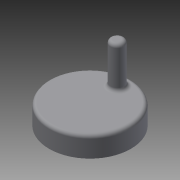
# Autodesk Inventor part: Handle
Saved by Autodesk Inventor 2014 (Build 180170000, 170)
## iProperties
Created: 2014-05-06
Part Number: Handle
Material: Generic
Document SubType Name: Modeling
Designer: Tristan Debrunner
Density: 1 g/cm^3
Appearance: Default
Author: Tristan Debrunner
Autodesk Inventor part; units mm, degrees
ref_plane "YZ Plane" through (0, 0, 0) normal (1, 0, 0) x (0, 1, 0)
ref_plane "XZ Plane" through (0, 0, 0) normal (0, 1, 0) x (-1, 0, 0)
ref_plane "XY Plane" through (0, 0, 0) normal (0, 0, 1) x (1, 0, 0)
sketch "Sketch1" plane through (0, 0, 0) normal (0, 1, 0) x (-1, 0, 0)
  circle A0 centre (0, 0) radius 38.1
  dimension "d0" = 76.2
  constraints: 1 centre point, 1 coincident
  measures "d0" diameter of A0
extrude "Extrusion1" add sketch "Sketch1" along normal blind 19.05
sketch "Sketch3" plane through (0, 0, 0) normal (0, -1, 0) x (1, 0, 0)
  circle A0 centre (0, 0) radius 38.1 projected
  line L0 (-9.271, 9.271) -> (9.271, 9.271)
  line L1 (9.271, 9.271) -> (9.271, -9.271)
  line L2 (9.271, -9.271) -> (-9.271, -9.271)
  line L3 (-9.271, -9.271) -> (-9.271, 9.271)
  line L4 (-9.271, 9.271) -> (9.271, -9.271) construction
  line L5 (9.271, 9.271) -> (-9.271, -9.271) construction
  dimension "d5" = 18.542
  dimension "d6" = 18.542
  constraints: 12 end point, 2 midpoint, 2 parallel, 1 horizontal, 1 perpendicular
  measures "d5" distance of L1.end L2.end
  measures "d6" distance of L0.end L1.end
extrude "Extrusion2" cut sketch "Sketch3" against normal blind 15.24 contours L0 L1 L2 L3
sketch "Sketch4" plane through (0, 19.05, 0) normal (0, 1, 0) x (1, 0, 0)
  circle A0 centre (0, 0) radius 38.1 projected
  line L0 (0, 0) -> (0, 25.4) construction
  circle A1 centre (0, 25.4) radius 6.35
  dimension "d9" = 25.4
  dimension "d10" = 12.7
  constraints: 2 end point, 1 centre point, 1 coincident, 1 vertical
  measures "d9" distance of L0.start L0.end
  measures "d10" diameter of A1
extrude "Extrusion3" add sketch "Sketch4" along normal blind 38.1 contours A1
fillet "Fillet1" radius 3.175 3 edges at (38.1, 19.05, 0) (-6.35, 19.05, -25.4) (-6.35, 57.15, -25.4)
body "Solid1"
